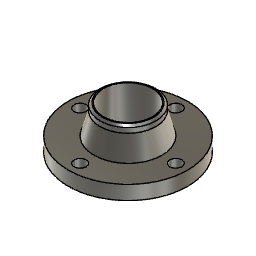
asme 3inch flange v3 (Autodesk Fusion 360 design; units mm, degrees)
Autodesk Fusion 360 part; units mm, degrees
note: some values were not read from the file. Set by a fixed rule: which sketch regions a step uses.
sketch "Sketch1" plane through (0, 0, 0) normal (0, 1, 0) x (1, 0, 0)
  line L0 (-15.2416, 0) -> (111.7584, 0)
  line L1 (48.2584, 0) -> (48.2584, -53.1739) construction
  line L2 (48.2584, 0) -> (48.2584, 47.0218) construction
  line L3 (111.7584, 0) -> (111.7584, -2)
  line L4 (111.7584, -2) -> (143.2584, -2)
  line L5 (143.2584, -2) -> (143.2584, -24.4)
  line L6 (143.2584, -24.4) -> (102.2584, -24.4)
  line L7 (48.2584, 0) -> (48.2584, -70)
  line L8 (48.2584, -70) -> (87.2184, -70)
  line L9 (48.2584, -70) -> (87.2184, -70)
  line L10 (48.2584, -70) -> (87.2184, -70)
  line L11 (87.2184, -70) -> (87.2184, 10) construction
  line L12 (87.2184, 10) -> (92.7084, 10) construction
  line L13 (92.7084, 10) -> (92.7084, -70) construction
  line L14 (92.7084, -70) -> (102.2584, -70) construction
  line L15 (102.2584, -70) -> (102.2584, 10) construction
  line L16 (102.2584, 10) -> (92.7084, 10) construction
  line L17 (87.2184, -70) -> (84.6384, -70) construction
  line L18 (92.7084, -59.1619) -> (102.2584, -24.4)
  line L19 (87.2184, -70) -> (88.8184, -70)
  line L20 (88.8184, -70) -> (92.7084, -67.0151)
  line L21 (88.8184, -70) -> (93.7216, -70) construction
  line L22 (92.7084, -67.0151) -> (92.7084, -59.1619)
  line L23 (87.2184, -70) -> (87.2184, 0)
  line L24 (48.2584, 0) -> (111.7584, 0)
  line L25 (124.4584, 0) -> (124.4584, -29) construction
  dimension "d1" = 127
  dimension "d2" = 2
  dimension "d3" = 22.4
  dimension "d4" = 31.5
  dimension "d5" = 70
  dimension "d6" = 38.96
  dimension "d7" = 44.45
  dimension "d11" = 9.55
  dimension "d13" = 1.6
  dimension "d14" = 37.5
  dimension "d21" = 76.2
  constraint midpoint L0 L1.start
  constraint perpendicular L0 L1
  constraint perpendicular L0 L3
  constraint perpendicular L3 L4
  constraint perpendicular L4 L5
  constraint perpendicular L3 L6
  constraint perpendicular L0 L7
  constraint perpendicular L7 L8
  constraint perpendicular L7 L9
  constraint perpendicular L7 L10
  constraint perpendicular L10 L11
  constraint perpendicular L11 L12
  constraint perpendicular L9 L13
  constraint perpendicular L14 L15
  constraint perpendicular L13 L16
  constraint horizontal L17
  constraint coincident L13 L18.start
  constraint perpendicular L11 L19
  constraint horizontal L21
  constraint coincident L13 L20.end
  constraint coincident L11 L23.end
  constraint coincident L0 L23.end
  constraint perpendicular L7 L24
  constraint perpendicular L24 L25
  measures "d1" distance of L0.start L0.end
  measures "d2" distance of L0.end L3.end
  measures "d3" distance of L4.end L5.end
  measures "d4" distance of L3.end L4.end
  measures "d5" distance of L1.start L7.end
  measures "d6" distance of L7.end L8.end
  measures "d7" distance of L7.end L13.end
  measures "d11" horizontal distance of L6.end L18.start
  measures "d13" distance of L8.end L19.end
  measures "d14" angle of L20 L21
  measures "d21" distance of L1.start L25.start
revolve "Revolve1" add sketch "Sketch1" angle 360 about axis through (48.2584, 0, 0) along (0, 0, 1) contours L0 L3 L4 L5 L6 L18 L19 L20 L22 L23 L24
sketch "Sketch2" plane through (0, 0, 24.4) normal (0, 0, 1) x (-1, 0, 0)
  circle A0 centre (-48.2584, 0) radius 95
  circle A1 centre (-48.2584, 0) radius 54
  line L0 (-143.2584, 0) -> (-102.2584, 0)
  line L1 (-102.2584, 0) -> (-114.9584, 0)
  line L2 (15.2416, 0) -> (-111.7584, 0)
  line L3 (-48.2584, 0) -> (-80, 0)
  line L4 (-48.2584, 0) -> (-124.4584, 0)
  circle A2 centre (-124.4584, 0) radius 9.525
  circle A3 centre (-48.2584, -76.2) radius 9.525
  circle A4 centre (27.9416, 0) radius 9.525
  circle A5 centre (-48.2584, 76.2) radius 9.525
  point P0 (-124.4584, 0)
  point P1 (-102.2584, 0)
  dimension "d22" = 12.7
  dimension "d23" = 76.2
  dimension "d24" = 19.05
  dimension "d26" = 360
  constraint coincident P1 L0.end
  constraint parallel L0 L1
  constraint coincident A0.centre A1.centre
  constraint coincident L2 L3.end
  constraint parallel L2 L4
  constraint coincident P0 L4.end
  measures "d22" distance of P1 L1.end
  measures "d23" distance of A0.centre P0
  measures "d24" diameter of A2
extrude "Extrude2" cut sketch "Sketch2" against normal blind 100 contours L0 L1 L4 A2 | L0 L1 L4 A2 | A3 | A4 | A5
